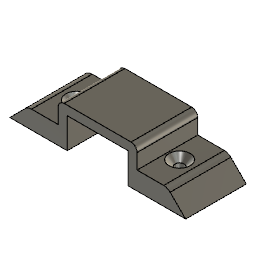
cable fastener (Autodesk Fusion 360 design; units mm, degrees)
part number: 2026-04-14-18-28-00-852
Autodesk Fusion 360 part; units mm, degrees
sketch "Sketch1" plane through (0, 0, 0) normal (0, 1, 0) x (1, 0, 0)
  line L0 (-10, 0) -> (-10, -10)
  line L1 (-10, -10) -> (10, -10)
  line L2 (10, -10) -> (10, 0)
  line L3 (10, 0) -> (13, 0)
  line L4 (13, 0) -> (13, -13)
  line L5 (13, -13) -> (-13, -13)
  line L6 (-13, -13) -> (-13, 0)
  line L7 (-13, 0) -> (-10, 0)
  line L8 (0, 0) -> (0, -10) construction
  line L9 (-13, -6) -> (-23, -6)
  line L10 (-23, -6) -> (-29, 0)
  line L11 (-29, 0) -> (-13, 0)
  line L12 (13, -6) -> (23, -6)
  line L13 (29, 0) -> (13, 0)
  line L14 (23, -6) -> (29, 0)
  dimension "d1" = 20
  dimension "d2" = 10
  dimension "d6" = 13
  dimension "d7" = 13
  dimension "d8" = 3
  dimension "d9" = 3
  dimension "d10" = 10
  dimension "d11" = 45
  dimension "d12" = 10
  constraint vertical L0
  constraint perpendicular L0 L1
  constraint perpendicular L1 L2
  constraint perpendicular L2 L3
  constraint perpendicular L3 L4
  constraint perpendicular L4 L5
  constraint perpendicular L3 L6
  constraint perpendicular L0 L7
  constraint coincident L8.start origin
  constraint midpoint L1 L8.end
  constraint perpendicular L1 L8
  constraint coincident L6 L9.start
  constraint perpendicular L6 L9
  constraint perpendicular L6 L11
  constraint symmetric L6.end L8 L3.end
  constraint symmetric L8 L9.start L12.start
  constraint symmetric L8 L9.end L12.end
  constraint symmetric L8 L10.end L13.start
  measures "d1" distance of L0.end L1.end
  measures "d2" distance of L0.start L0.end
  measures "d6" distance of L5.end L6.end
  measures "d7" distance of L3.end L4.end
  measures "d8" distance of L0.start L6.end
  measures "d9" distance of L2.end L3.end
  measures "d10" distance of L8.start L8.end
  measures "d11" angle of L10 L11
  measures "d12" distance of L9.start L9.end
extrude "Extrude1" add sketch "Sketch1" along normal blind 20
fillet "Fillet1" radius 3 1 edges at (-23, 10, 6)
mirror "Mirror1" about plane through (0, 0, 0) normal (1, 0, 0) of 1 faces at (-22.0188, 6.6667, 5.9886)
fillet "Fillet2" radius 2 1 edges at (-13, 10, 13)
mirror "Mirror2" about plane through (0, 0, 0) normal (1, 0, 0) of 1 faces at (-11.1901, 6.6667, 12.9909)
sketch "Sketch2" plane through (0, 0, 13) normal (0, 0, 1) x (-1, 0, 0)
  line L0 (-11, 0) -> (-11, -20)
  line L1 (-11, -20) -> (11, -20)
  line L2 (11, -20) -> (11, 0)
  line L3 (11, 0) -> (-11, 0)
  line L4 (0, 0) -> (0, -10) construction
  line L5 (0, -10) -> (17, -10) construction
  circle A0 centre (17, -10) radius 1.5
  circle A1 centre (-17, -10) radius 1.5
  dimension "d24" = 10
  dimension "d25" = 17
  dimension "d26" = 3
  constraint coincident L4.start origin
  constraint perpendicular L3 L4
  constraint perpendicular L4 L5
  constraint coincident L5.end A0.centre
  constraint symmetric L4 A0 A1
  measures "d24" distance of L4.start L4.end
  measures "d25" distance of L4.end L5.end
  measures "d26" diameter of A0
extrude "Extrude3" cut sketch "Sketch2" against normal blind 22 contours A0 | A1
chamfer "Chamfer2" distance 2 angle 45 2 edges at (-15.6015, 9.4576, 6) (18.3985, 9.4576, 6)
equation "d1 = width_inner"
equation "d2 = height_inner"
equation "thickness = 3 mm"
equation "height_inner = 10 mm"
equation "width_inner = 20 mm"
equation "d6 = height_inner + thickness"
equation "d7 = height_inner + thickness"
equation "d8 = thickness"
equation "d9 = thickness"
equation "d10 = height_inner"
equation "d13 = body_width"
equation "body_width = 20 mm"
equation "d24 = body_width / 2"
equation "d25 = width_inner / 2 + thickness + 4 mm"
